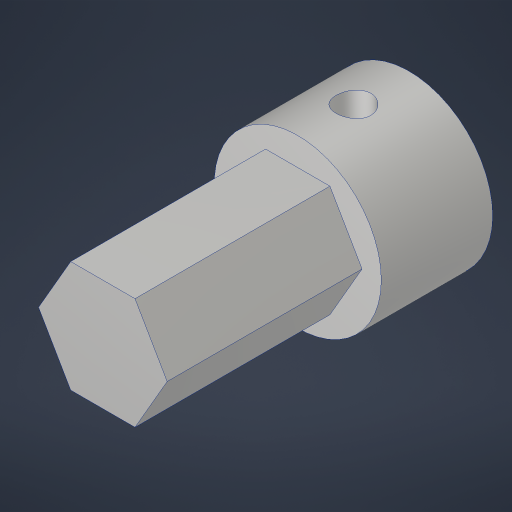
# Autodesk Inventor part: CL7-016
Saved by Autodesk Inventor 2023.4 (Build 274418000, 418)
## iProperties
Created: 2025-03-19
Part Number: CL7-016
Material: Aluminum 6061
Document SubType Name: Modeling
Designer: slick
Density: 2.7 g/cm^3
Appearance: Aluminum - Flat
Author: slick
Autodesk Inventor part; units mm, degrees
ref_plane "YZ Plane" through (0, 0, 0) normal (1, 0, 0) x (0, 1, 0)
ref_plane "XZ Plane" through (0, 0, 0) normal (0, 1, 0) x (-1, 0, 0)
ref_plane "XY Plane" through (0, 0, 0) normal (0, 0, 1) x (1, 0, 0)
sketch "Sketch1" plane through (0, 0, 0) normal (0, 0, 1) x (1, 0, 0)
  circle A0 centre (0, 0) radius 9.525
  dimension "d0" = 19.05
  constraints: 1 centre point, 1 coincident
  measures "d0" diameter of A0
extrude "Extrusion1" add sketch "Sketch1" along normal blind 34.925
sketch "Sketch2" plane through (0, 0, 34.925) normal (0, 0, 1) x (1, 0, 0)
  line L0 (-3.6662, 6.35) -> (3.6662, 6.35)
  line L1 (3.6662, 6.35) -> (7.3323, 0)
  line L2 (7.3323, 0) -> (3.6662, -6.35)
  line L3 (3.6662, -6.35) -> (-3.6662, -6.35)
  line L4 (-3.6662, -6.35) -> (-7.3323, 0)
  line L5 (-7.3323, 0) -> (-3.6662, 6.35)
  circle A0 centre (0, 0) radius 9.525 projected
  dimension "d3" = 12.7
  constraints: 12 end point, 1 coincident, 1 horizontal, 13 other
  measures "d3" distance between parallel lines of L3 L0
extrude "Extrusion2" cut sketch "Sketch2" against normal blind 22.225
sketch "Sketch3" plane through (0, 0, 0) normal (0, 1, 0) x (-1, 0, 0)
  line L0 (9.525, 0) -> (-9.525, 0) construction
  line L1 (3.6662, 34.925) -> (-3.6662, 34.925) construction
  point P0 (0, 0)
  point P1 (0, 6.35)
  point P2 (0, 34.925)
  dimension "d6" = 6.35
  constraints: 1 midpoint, 1 vertical alignment
  measures "d6" distance from line of L0 point (0, 6.35)
hole "Hole1" at (0, 0, 6.35) direction (0, -1, 0) diameter 3.9624 end through all start extended yes thread size "10-32 UNF" class "2B" standard "ANSI Unified Screw Threads"
body "Solid1"
